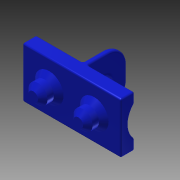
# Autodesk Inventor part: Leg Joint
Saved by Autodesk Inventor 2013 (Build 170138000, 138)
## iProperties
Created: 2013-09-06
Part Number: Leg Joint
Material: Generic
Document SubType Name: Modeling
Designer: 200395375
Density: 1 g/cm^3
Mass: 0.301248 g
Surface Area: 4.88674 cm^2
Volume: 0.301248 cm^3
Author: 200395375
Autodesk Inventor part; units mm, degrees
ref_plane "YZ Plane" through (0, 0, 0) normal (1, 0, 0) x (0, 1, 0)
ref_plane "XZ Plane" through (0, 0, 0) normal (0, 1, 0) x (-1, 0, 0)
ref_plane "XY Plane" through (0, 0, 0) normal (0, 0, 1) x (1, 0, 0)
sketch "Sketch1" plane through (0, 0, 0) normal (0, 1, 0) x (-1, 0, 0)
  line L0 (0, 0) -> (15.44, 0)
  line L1 (15.44, 0) -> (15.44, -8)
  line L2 (15.44, -8) -> (0, -8)
  line L3 (0, -8) -> (0, 0)
  dimension "d0" = 15.44
  dimension "d1" = 8
  constraints: 8 end point, 2 parallel, 1 horizontal, 1 perpendicular
  measures "d0" distance of L1.end L2.end
  measures "d1" distance of L0.end L1.end
extrude "Extrusion1" add sketch "Sketch1" along normal blind 2.15
sketch "Sketch2" plane through (0, 2.15, 0) normal (0, 1, 0) x (1, 0, 0)
  line L0 (-15.44, 0) -> (0, 0) projected
  line L1 (0, 8) -> (-15.44, 8) projected
  line L2 (-7.72, 8) -> (-7.32, 8)
  line L3 (-7.32, 8) -> (-8.12, 8)
  line L4 (-8.12, 8) -> (-8.12, 0)
  line L5 (-8.12, 0) -> (-7.32, 0)
  line L6 (-7.32, 0) -> (-7.32, 8)
  dimension "d4" = 0.4
  dimension "d5" = 0.8
  constraints: 10 end point, 2 parallel, 2 point on line, 1 horizontal, 1 midpoint, 1 perpendicular
  measures "d4" distance of L2.start L2.end
  measures "d5" distance of L5.end L4.end
extrude "Extrusion2" add sketch "Sketch2" along normal blind 6.1
sketch "Sketch3" plane through (-7.32, 2.15, 0) normal (1, 0, 0) x (0, 0, -1)
  line L0 (0, 6.1) -> (8, 6.1) projected
  circle A0 centre (4, 2.56) radius 3.54
  circle A1 centre (4, 2.56) radius 0.75
  point P0 (0, -2.15)
  dimension "d8" = 7.08
  dimension "d11" = 1.5
  constraints: 2 centre point, 1 coincident, 1 tangent
  measures "d8" diameter of A0
  measures "d11" diameter of A1
extrude "Extrusion3" add sketch "Sketch3" along normal blind 3 contours A1
sketch "Sketch4" plane through (-8.12, 2.15, -8) normal (-1, 0, 0) x (0, 0, 1)
  line L0 (0, 6.1) -> (8, 6.1) projected
  circle A0 centre (4, 2.56) radius 3.54
  circle A1 centre (4, 2.56) radius 0.75
  point P0 (8, -2.15)
  dimension "d14" = 7.08
  dimension "d16" = 1.5
  constraints: 2 centre point, 1 coincident, 1 tangent
  measures "d14" diameter of A0
  measures "d16" diameter of A1
extrude "Extrusion4" add sketch "Sketch4" along normal blind 3 contours A1
fillet "Fillet1" radius 3 2 edges at (-7.72, 8.25, -8) (-7.72, 8.25, 0)
sketch "Sketch6" plane through (0, 0, 0) normal (1, 0, 0) x (0, 0, -1)
  circle A0 centre (4, 4.71) radius 3.505
  circle A1 centre (4, 4.71) radius 0.75 projected
  dimension "d22" = 7.01
  constraints: 1 centre point, 1 concentric
  measures "d22" diameter of A0
extrude "Extrusion5" cut sketch "Sketch6" against normal up to surface (7.32 mm away)
sketch "Sketch7" plane through (-15.44, 0, -8) normal (-1, 0, 0) x (0, 0, 1)
  circle A0 centre (4, 4.71) radius 3.54
  circle A1 centre (4, 4.71) radius 0.75 projected
  dimension "d25" = 7.08
  constraints: 1 centre point, 1 concentric
  measures "d25" diameter of A0
extrude "Extrusion6" cut sketch "Sketch7" against normal up to surface (7.32 mm away)
fillet "Fillet2" radius 0.25 38 edges at (-7.32, 7.3713, -7.1213) (-7.32, 3.7, -8) (-7.32, 8.25, -4) (-7.32, 7.3713, -0.8787) (-7.32, 3.7, 0) (-8.12, 8.25, -4) (-8.12, 7.3713, -0.8787) (-8.12, 3.7, 0) (-8.12, 3.7, -8) (-8.12, 7.3713, -7.1213) (-7.32, 2.15, -7.197) (-8.12, 2.15, -7.2225) (-7.32, 2.15, -0.803) (-8.12, 2.15, -0.7775) (-3.66, 2.15, -8) (-11.78, 2.15, -8) (-3.66, 2.15, 0) (-11.78, 2.15, 0) (-15.44, 2.15, -7.2225) (-15.44, 1.17, -4) (-15.44, 2.15, -0.7775) (-11.78, 2.15, -1.555) (-11.78, 2.15, -6.445) (-7.72, 0, 0) (-3.66, 2.15, -1.606) (-3.66, 2.15, -6.394) (-7.72, 0, -8) (0, 1.205, -4) (0, 2.15, -7.197) (0, 2.15, -0.803) (0, 0, -4) (-15.44, 0, -4) (-8.12, 1.17, -4) (-7.32, 1.205, -4) (-15.44, 1.075, 0) (-15.44, 1.075, -8) (0, 1.075, -8) (0, 1.075, 0)
fillet "Fillet3" radius 0.75 4 edges at (-7.32, 4.71, -3.25) (-4.32, 4.71, -3.25) (-8.12, 4.71, -4.75) (-11.12, 4.71, -4.75)
sketch "Sketch8" plane through (0, 0, 0) normal (0, -1, 0) x (1, 0, 0)
  circle A0 centre (-11.254, -4) radius 1.5
  circle A1 centre (-4.186, -4) radius 1.5
  line L0 (-0.25, 0) -> (-15.19, 0) projected
  line L1 (-15.44, -0.25) -> (-15.44, -7.75) projected
  line L2 (-15.19, -0.25) -> (-0.25, -0.25) projected
  line L3 (-0.25, -7.75) -> (-15.19, -7.75) projected
  line L4 (-7.72, -0.25) -> (-7.72, -7.75)
  point P0 (0, 0)
  dimension "d30" = 3
  dimension "d31" = 3
  dimension "d40" = 7.068
  constraints: 2 centre point, 2 end point, 2 midpoint
  measures "d30" diameter of A0
  measures "d31" diameter of A1
  measures "d40" distance of A1.centre A0.centre
extrude "Extrusion7" add sketch "Sketch8" along normal blind 2.5
chamfer "Chamfer1" distance 0.75 angle 45 4 edges at (-5.686, 0, -4) (-5.686, -2.5, -4) (-12.754, 0, -4) (-12.754, -2.5, -4)
body "Solid1"
